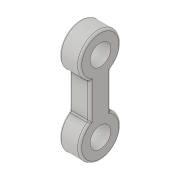
# Autodesk Inventor part: Arm
Saved by Autodesk Inventor 2017 (Build 210142000, 142)
## iProperties
Created: 2016-07-28
Part Number: Arm
Material: Generic
Document SubType Name: Modeling
Designer: Tutorial Books
Density: 1 g/cm^3
Appearance: Default
Author: Tutorial Books
Autodesk Inventor part; units mm, degrees
ref_plane "YZ Plane" through (0, 0, 0) normal (1, 0, 0) x (0, 1, 0)
ref_plane "XZ Plane" through (0, 0, 0) normal (0, 1, 0) x (-1, 0, 0)
ref_plane "XY Plane" through (0, 0, 0) normal (0, 0, 1) x (1, 0, 0)
sketch "Sketch1" plane through (0, 0, 0) normal (1, 0, 0) x (0, 1, 0)
  circle A0 centre (35.052, 0) radius 5.08
  arc A1 (26.2532, -5.08) -> (26.2532, 5.08) centre (35.052, 0) ccw
  circle A2 centre (0, 0) radius 5.08
  arc A3 (8.7988, 5.08) -> (8.7988, -5.08) centre (0, 0) ccw
  line L0 (26.2532, 5.08) -> (8.7988, 5.08)
  line L1 (26.2532, -5.08) -> (8.7988, -5.08)
  dimension "d0" = 10.16
  dimension "d1" = 10.16
  dimension "d2" = 35.052
  dimension "d3" = 10.16
  dimension "d4" = 5.08
  constraints: 4 centre point, 4 end point, 4 point on circle, 3 coincident, 2 equal radius, 2 horizontal, 1 horizontal alignment
  measures "d0" radius of A1
  measures "d1" diameter of A0
  measures "d2" distance of A2.centre A0.centre
  measures "d3" distance between parallel lines of L1 L0
  measures "d4" distance from line of point (0, 0) L0
extrude "Extrusion1" add sketch "Sketch1" along normal mid plane 10.16
fillet "Fillet1" radius 1.016 8 edges at (5.08, 45.212, 0) (5.08, 17.526, -5.08) (5.08, -10.16, 0) (5.08, 17.526, 5.08) (-5.08, 45.212, 0) (-5.08, 17.526, -5.08) (-5.08, -10.16, 0) (-5.08, 17.526, 5.08)
fillet "Fillet2" radius 1.016 12 edges at (4.8026, 26.4389, 4.7617) (-4.8026, 26.4389, 4.7617) (0, 26.2532, 5.08) (-4.8026, 8.6131, 4.7617) (4.8026, 8.6131, 4.7617) (0, 8.7988, 5.08) (-4.8026, 26.4389, -4.7617) (4.8026, 26.4389, -4.7617) (0, 26.2532, -5.08) (-4.8026, 8.6131, -4.7617) (4.8026, 8.6131, -4.7617) (0, 8.7988, -5.08)
body "Solid1"
